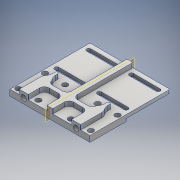
# Autodesk Inventor part: Portal-Column-v2-base
Saved by Autodesk Inventor 2016 (Build 200138000, 138)
## iProperties
Created: 2015-10-23
Part Number: Portal-Column-v2-base
Material: Aluminum 6061
Document SubType Name: Modeling
Designer: as
Density: 2.7 g/cm^3
Appearance: Aluminum - Flat
Mass: 74.5293 g
Surface Area: 100.965 cm^2
Volume: 27.6034 cm^3
Author: as
Autodesk Inventor part; units mm, degrees
ref_plane "YZ Plane" through (0, 0, 0) normal (1, 0, 0) x (0, 1, 0)
ref_plane "XZ Plane" through (0, 0, 0) normal (0, 1, 0) x (-1, 0, 0)
ref_plane "XY Plane" through (0, 0, 0) normal (0, 0, 1) x (1, 0, 0)
sketch "Sketch1" plane through (0, 0, 0) normal (0, 0, 1) x (1, 0, 0)
  line L0 (10.3, -7.5) -> (-10.3, -7.5) projected
  line L1 (10.3, -7.5) -> (-49.7, -7.5)
  line L2 (-49.7, -7.5) -> (-49.7, 52.5)
  line L3 (-49.7, 52.5) -> (10.3, 52.5)
  line L4 (10.3, 52.5) -> (10.3, -7.5)
  point P0 (0, 0)
  dimension "d0" = 60
  dimension "d1" = 60
  constraints: 8 end point, 2 parallel, 1 horizontal, 1 perpendicular
  measures "d0" distance of L2.end L3.end
  measures "d1" distance of L1.end L2.end
extrude "Extrusion1" add sketch "Sketch1" along normal blind 8
sketch "Sketch2" plane through (0, 0, 8) normal (0, 0, 1) x (1, 0, 0)
  line L0 (-687.1207, 43.5) -> (-687.1207, 27.5) projected
  line L1 (32.8793, 27.5) -> (-687.1207, 27.5) projected
  line L2 (32.8793, 43.5) -> (32.8793, 27.5) projected
  line L3 (32.8793, 43.5) -> (-687.1207, 43.5) projected
  circle A0 centre (7.5, -4) radius 1.2295 projected
  circle A1 centre (-7.5, -4) radius 1.2295 projected
  circle A2 centre (7.5, 16) radius 1.2295 projected
  circle A3 centre (-7.5, 16) radius 1.2295 projected
  point P0 (0, 0)
hole "Hole1" at (7.5, -4, 8) at (-7.5, -4, 8) at (7.5, 16, 8) at (-7.5, 16, 8) direction (0, 0, -1) diameter 4 end through all
ref_plane "Work Plane1" through (-19.7, -7.5, 0) normal (1, 0, 0) x (0, 0, -1)
mirror "Mirror1" about plane through (-19.7, -7.5, 0) normal (1, 0, 0) of "Hole1"
sketch "Sketch3" plane through (-49.7, -7.5, 0) normal (0, -1, 0) x (1, 0, 0)
  line L0 (44.2, 0) -> (44.2, 8) projected
  line L1 (55.2, 0) -> (55.2, 8) projected
  line L2 (0, 8) -> (60, 8) construction
  line L3 (60, 0) -> (0, 0) construction
  line L4 (49.7, 4) -> (44.2, 4) construction
  line L5 (49.7, 4) -> (55.2, 4) construction
  line L6 (49.7, 4) -> (49.7, 0) construction
  line L7 (49.7, 4) -> (49.7, 8) construction
  constraints: 8 end point, 3 point on line, 2 collinear, 2 midpoint, 1 perpendicular
hole "Hole2" at (0, -7.5, 4) direction (0, 1, 0) diameter 4.134 depth 14.2 tip angle 118 thread size "M5x0.8" class "6H" standard "ISO Metric profile"
mirror "Mirror2" about plane through (-19.7, -7.5, 0) normal (1, 0, 0) of "Hole2"
sketch "Sketch5" plane through (0, 0, 8) normal (0, 0, 1) x (1, 0, 0)
  line L0 (10.3, -7.5) -> (3.3, -7.5)
  line L1 (3.3, -7.5) -> (3.3, 41.5)
  line L2 (3.3, 52.5) -> (10.3, 52.5)
  line L3 (10.3, 52.5) -> (10.3, -7.5)
  line L4 (10.3, -7.5) -> (10.3, 52.5) projected
  line L5 (-49.7, -7.5) -> (10.3, -7.5) projected
  line L6 (10.3, -7.5) -> (-49.7, -7.5) projected
  line L7 (-3.5, -7.5) -> (-17.5, -7.5)
  line L8 (-17.5, -7.5) -> (-17.5, 52.5)
  line L9 (-17.5, 52.5) -> (-3.5, 52.5)
  line L10 (-3.5, 52.5) -> (-3.5, -7.5)
  circle A0 centre (-7.5, -4) radius 2 projected
  line L11 (3.3, 52.5) -> (-3.5, 52.5)
  line L12 (-3.5, 52.5) -> (-3.5, 41.5)
  line L13 (-3.5, 41.5) -> (3.3, 41.5)
  line L14 (3.3, 41.5) -> (3.3, 52.5)
  point P0 (0, 0)
  dimension "d28" = 7
  dimension "d29" = 60
  dimension "d30" = 14
  dimension "d31" = 60
  dimension "d32" = 4
  dimension "d33" = 11
  constraints: 24 end point, 7 parallel, 3 horizontal, 3 perpendicular, 2 collinear, 2 point on line
  measures "d28" distance of L2.start L2.end
  measures "d29" distance of L0.end L2.start
  measures "d30" distance of L8.end L9.end
  measures "d31" distance of L7.end L8.end
  measures "d32" distance from line of A0.centre L10
  measures "d33" distance of L12.end L11.end
extrude "Extrusion2" cut sketch "Sketch5" against normal blind 3.5 contours L0 L1 L14 L2 L3 | L5 L8 L9 L10
sketch "Sketch8" plane through (0, 0, 8) normal (0, 0, 1) x (1, 0, 0)
  line L0 (-3.5, 52.5) -> (-3.5, -7.5) construction
  line L1 (3.3, 52.5) -> (-3.5, 52.5) construction
  line L2 (-3.5, 10.5) -> (-1.2, 10.5)
  line L3 (-1.2, 10.5) -> (-1.2, 52.5)
  line L4 (-1.2, 52.5) -> (-3.5, 52.5)
  line L5 (-3.5, 52.5) -> (-3.5, 10.5)
  line L6 (3.3, 10.5) -> (1, 10.5)
  line L7 (1, 10.5) -> (1, 52.5)
  line L8 (1, 52.5) -> (3.3, 52.5)
  line L9 (3.3, 52.5) -> (3.3, 10.5)
  line L10 (3.3, -7.5) -> (3.3, 52.5) projected
  line L11 (-1.2, 18) -> (1, 18)
  line L12 (-1.2, 52.5) -> (1, 52.5)
  point P0 (0, 0)
  dimension "d48" = 2.3
  dimension "d49" = 2.3
  constraints: 20 end point, 5 point on line, 4 parallel, 3 perpendicular, 2 collinear, 2 horizontal
  measures "d48" distance of L4.end L3.end
  measures "d49" distance of L7.end L8.end
extrude "Extrusion5" cut sketch "Sketch8" against normal blind 3.5
fillet "Fillet5" radius 6 4 edges at (1, 10.5, 6.25) (-1.2, 10.5, 6.25) (-3.5, 10.5, 6.25) (3.3, 10.5, 6.25)
sketch "Sketch6" plane through (0, 0, 4.5) normal (0, 0, 1) x (1, 0, 0)
  line L0 (-3.5, 52.5) -> (-3.5, -7.5) projected
  line L1 (-17.5, -7.5) -> (-17.5, 52.5) projected
  line L2 (-3.5, 4.5) -> (-17.5, 4.5)
  line L3 (-17.5, 4.5) -> (-17.5, 7.5)
  line L4 (-17.5, 7.5) -> (-3.5, 7.5)
  line L5 (-3.5, 7.5) -> (-3.5, 4.5)
  line L6 (-3.5, -7.5) -> (-17.5, -7.5) projected
  point P0 (0, 0)
  point P1 (-3.5, 11.5)
  point P2 (-17.5, 22.5)
  dimension "d37" = 3
  dimension "d47" = 12
  constraints: 8 end point, 2 parallel, 2 point on line, 1 horizontal, 1 perpendicular
  measures "d37" distance of L2.end L3.end
  measures "d47" distance between parallel lines of L6 L2
extrude "Extrusion3" add sketch "Sketch6" along normal blind 3.5 contours L0 L2 L1 L4
fillet "Fillet1" radius 3.5 4 edges at (-3.5, 7.5, 6.25) (-17.5, 7.5, 6.25) (-17.5, 4.5, 6.25) (-3.5, 4.5, 6.25)
fillet "Fillet6" radius 1.1 2 edges at (1, 18, 6.25) (-1.2, 18, 6.25)
fillet "Fillet3" radius 0.2 3 edges at (3.3, -7.5, 6.25) (-3.5, -7.5, 6.25) (-17.5, -7.5, 6.25)
mirror "Mirror3" about plane through (-19.7, -7.5, 0) normal (1, 0, 0) of "Extrusion2", "Extrusion3", "Fillet1", "Fillet3", "Extrusion5", "Fillet5", "Fillet6"
sketch "Sketch7" plane through (0, 0, 0) normal (0, 0, -1) x (-1, 0, 0)
  line L0 (-10.3, 52.5) -> (-10.3, -7.5) projected
  line L1 (-10.3, 52.5) -> (49.7, 52.5)
  line L2 (49.7, 52.5) -> (49.7, 19.5)
  line L3 (49.7, 19.5) -> (-10.3, 19.5)
  line L4 (-10.3, 19.5) -> (-10.3, 52.5)
  point P0 (0, 0)
  dimension "d42" = 60
  dimension "d43" = 33
  constraints: 8 end point, 2 parallel, 1 horizontal, 1 perpendicular
  measures "d42" distance of L2.end L3.end
  measures "d43" distance of L1.end L2.end
extrude "Extrusion4" cut sketch "Sketch7" against normal blind 2
sketch "Sketch9" plane through (0, 0, 2) normal (0, 0, -1) x (-1, 0, 0)
  line L0 (-6.3, 23.5) -> (13.7, 23.5) construction
  line L1 (-6.3, 21.95) -> (13.7, 21.95)
  line L2 (13.7, 25.05) -> (-6.3, 25.05)
  arc A0 (-6.3, 25.05) -> (-6.3, 21.95) centre (-6.3, 23.5) ccw
  arc A1 (13.7, 21.95) -> (13.7, 25.05) centre (13.7, 23.5) ccw
  line L3 (-11.991, 23.5) -> (58.009, 23.5) construction
  line L4 (49.7, 19.5) -> (-10.3, 19.5) construction
  line L5 (-11.991, 23.5) -> (58.009, 23.5) construction
  line L6 (58.009, 23.5) -> (58.009, 43.5) construction
  line L7 (58.009, 43.5) -> (-11.991, 43.5) construction
  line L8 (-10.3, 19.5) -> (-10.3, 52.5) projected
  point P0 (0, 0)
  point P1 (3.7, 23.5)
  dimension "d53" = 20
  dimension "d54" = 3.1
  dimension "d57" = 70
  dimension "d58" = 0
  dimension "d59" = 20
  dimension "d60" = 70
  dimension "d62" = 4
  dimension "d63" = 4
  constraints: 16 end point, 4 point on circle, 4 tangent, 2 centre point, 2 horizontal, 2 parallel, 2 perpendicular, 1 collinear, 1 midpoint, 1 point on line
  measures "d53" distance of L0.start L0.end
  measures "d54" diameter of A1
  measures "d57" distance of L3.start L3.end
  measures "d58" distance between parallel lines of L3 L5
  measures "d59" distance of L3.end L6.end
  measures "d60" distance of L6.end L7.end
  measures "d62" distance from line of L8 L0.start
  measures "d63" distance from line of L4 point (3.7, 23.5)
extrude "Extrusion6" cut sketch "Sketch9" against normal through all
pattern_linear "Rectangular Pattern1" count 2 spacing 24 along (0, 1, 0) of "Extrusion6"
mirror "Mirror4" about plane through (-19.7, -7.5, 0) normal (1, 0, 0) of "Extrusion6", "Rectangular Pattern1"
fillet "Fillet7" radius 1.1 4 edges at (10.3, 52.5, 3.25) (-49.7, 52.5, 3.25) (-17.5, 52.5, 6.25) (-21.9, 52.5, 6.25)
equation "\"d49\" = d48"
body "Solid1"
